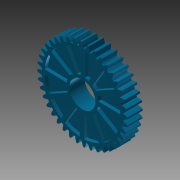
# Autodesk Inventor part: 12-0040_Gear
Saved by Autodesk Inventor 2015 SP1 (Build 190203100, 203)
## iProperties
Category: Gear Kit
Company: Autodesk Inc.
Created: 2014-11-29
Part Number: 12-0040_Gear
Material: Polystyrene, High Impact
Document SubType Name: Modeling
Designer: Matrix
Density: 1.022 g/cm^3
Appearance: Sky Blue Dark
Catalog Web Link: http://matrixrobotics.com/
Vendor: Matrix
Author: Autodesk Inc.
Autodesk Inventor part; units mm, degrees
ref_plane "YZ Plane" through (0, 0, 0) normal (1, 0, 0) x (0, 1, 0)
ref_plane "XZ Plane" through (0, 0, 0) normal (0, 1, 0) x (-1, 0, 0)
sketch "Sketch1" plane through (0, 0, 0) normal (0, 1, 0) x (-1, 0, 0)
  line L0 (9.9681, 15.9078) -> (10.1982, 16.6846)
  arc A0 (10.1982, 16.6846) -> (10.2097, 16.7356) centre (9.8146, 16.7982) ccw
  line L1 (10.2097, 16.7356) -> (10.3968, 17.917)
  arc A1 (10.3968, 17.917) -> (10.2983, 18.1191) centre (10.2032, 17.9477) ccw
  line L2 (9.9086, 18.3351) -> (10.2983, 18.1191)
  arc A2 (9.9086, 18.3351) -> (9.685, 18.3116) centre (9.8136, 18.1636) ccw
  line L3 (9.685, 18.3116) -> (8.7823, 17.5268)
  arc A3 (8.7823, 17.5268) -> (8.7451, 17.49) centre (9.0447, 17.225) ccw
  line L4 (8.7451, 17.49) -> (8.2083, 16.8833)
  arc A4 (8.0902, 16.8594) -> (8.2083, 16.8833) centre (8.1334, 16.9495) ccw
  arc A5 (8.0902, 16.8594) -> (7.4163, 17.1665) centre (0, 0) ccw
  arc A6 (7.3568, 17.2713) -> (7.4163, 17.1665) centre (7.456, 17.2583) ccw
  line L5 (7.3568, 17.2713) -> (7.466, 18.1005)
  line L6 (7.466, 18.1005) -> (7.466, 19.3228)
  arc A7 (7.466, 19.3228) -> (7.337, 19.507) centre (7.27, 19.3228) ccw
  line L7 (7.337, 19.507) -> (6.9184, 19.6594)
  arc A8 (6.9184, 19.6594) -> (6.7012, 19.6012) centre (6.8513, 19.4752) ccw
  line L8 (6.7012, 19.6012) -> (5.9155, 18.6648)
  line L9 (5.9155, 18.6648) -> (5.4661, 17.9595)
  arc A9 (5.3532, 17.9174) -> (5.4661, 17.9595) centre (5.3818, 18.0132) ccw
  arc A10 (5.3532, 17.9174) -> (4.6396, 18.1153) centre (0, 0) ccw
  arc A11 (4.5644, 18.2096) -> (4.6396, 18.1153) centre (4.6644, 18.2122) ccw
  line L10 (4.5644, 18.2096) -> (4.5425, 19.0456)
  line L11 (4.5425, 19.0456) -> (4.3513, 20.2529)
  arc A12 (4.3513, 20.2529) -> (4.1951, 20.4146) centre (4.1577, 20.2222) ccw
  line L12 (4.1951, 20.4146) -> (3.7578, 20.4996)
  arc A13 (3.7578, 20.4996) -> (3.5524, 20.4082) centre (3.7204, 20.3072) ccw
  line L13 (3.5524, 20.4082) -> (2.9228, 19.3604)
  line L14 (2.9228, 19.3604) -> (2.5894, 18.5935)
  arc A14 (2.4844, 18.5342) -> (2.5894, 18.5935) centre (2.4977, 18.6333) ccw
  arc A15 (2.4844, 18.5342) -> (1.7486, 18.6181) centre (0, 0) ccw
  arc A16 (1.6596, 18.6994) -> (1.7486, 18.6181) centre (1.7579, 18.7176) ccw
  line L15 (1.6596, 18.6994) -> (1.5072, 19.5217)
  line L16 (1.5072, 19.5217) -> (1.1295, 20.6842)
  arc A17 (1.1295, 20.6842) -> (0.9499, 20.8195) centre (0.9431, 20.6237) ccw
  line L17 (0.9499, 20.8195) -> (0.5047, 20.8351)
  arc A18 (0.5047, 20.8351) -> (0.3161, 20.7126) centre (0.4978, 20.6392) ccw
  line L18 (0.3161, 20.7126) -> (-0.1418, 19.5793)
  line L19 (-0.1418, 19.5793) -> (-0.3512, 18.7696)
  arc A19 (-0.4456, 18.6947) -> (-0.3512, 18.7696) centre (-0.448, 18.7947) ccw
  arc A20 (-0.4456, 18.6947) -> (-1.1854, 18.6624) centre (0, 0) ccw
  arc A21 (-1.286, 18.7288) -> (-1.1854, 18.6624) centre (-1.1918, 18.7622) ccw
  line L20 (-1.286, 18.7288) -> (-1.5652, 19.5171)
  line L21 (-1.5652, 19.5171) -> (-2.1201, 20.6063)
  arc A22 (-2.1201, 20.6063) -> (-2.3187, 20.7118) centre (-2.2948, 20.5173) ccw
  line L22 (-2.3187, 20.7118) -> (-2.7609, 20.6575)
  arc A23 (-2.7609, 20.6575) -> (-2.9279, 20.5071) centre (-2.737, 20.463) ccw
  line L23 (-2.9279, 20.5071) -> (-3.2029, 19.3161)
  line L24 (-3.2029, 19.3161) -> (-3.2831, 18.4836)
  arc A24 (-3.3646, 18.3948) -> (-3.2831, 18.4836) centre (-3.3826, 18.4932) ccw
  arc A25 (-3.3646, 18.3948) -> (-4.0903, 18.2472) centre (0, 0) ccw
  arc A26 (-4.2, 18.297) -> (-4.0903, 18.2472) centre (-4.1122, 18.3448) ccw
  line L25 (-4.2, 18.297) -> (-4.5991, 19.032)
  line L26 (-4.5991, 19.032) -> (-5.3176, 20.0209)
  arc A27 (-5.3176, 20.0209) -> (-5.5302, 20.0941) centre (-5.4761, 19.9057) ccw
  line L27 (-5.5302, 20.0941) -> (-5.9584, 19.9713)
  arc A28 (-5.9584, 19.9713) -> (-6.0999, 19.7966) centre (-5.9044, 19.7829) ccw
  line L28 (-6.0999, 19.7966) -> (-6.1852, 18.5772)
  line L29 (-6.1852, 18.5772) -> (-6.1341, 17.7425)
  arc A29 (-6.2008, 17.642) -> (-6.1341, 17.7425) centre (-6.2339, 17.7363) ccw
  arc A30 (-6.2008, 17.642) -> (-6.8944, 17.3827) centre (0, 0) ccw
  arc A31 (-7.0106, 17.4147) -> (-6.8944, 17.3827) centre (-6.9313, 17.4756) ccw
  line L30 (-7.0106, 17.4147) -> (-7.5197, 18.0782)
  line L31 (-7.5197, 18.0782) -> (-8.384, 18.9426)
  arc A32 (-8.384, 18.9426) -> (-8.6055, 18.9816) centre (-8.5226, 18.804) ccw
  line L32 (-8.6055, 18.9816) -> (-9.0093, 18.7933)
  arc A33 (-9.0093, 18.7933) -> (-9.1217, 18.5986) centre (-8.9264, 18.6157) ccw
  line L33 (-9.1217, 18.5986) -> (-9.0151, 17.3809)
  line L34 (-9.0151, 17.3809) -> (-8.8341, 16.5644)
  arc A34 (-8.8843, 16.4548) -> (-8.8341, 16.5644) centre (-8.9318, 16.5428) ccw
  arc A35 (-8.8843, 16.4548) -> (-9.5288, 16.0901) centre (0, 0) ccw
  arc A36 (-9.6486, 16.1036) -> (-9.5288, 16.0901) centre (-9.5797, 16.1762) ccw
  line L35 (-9.6486, 16.1036) -> (-10.2552, 16.6793)
  line L36 (-10.2552, 16.6793) -> (-11.2441, 17.3978)
  arc A37 (-11.2441, 17.3978) -> (-11.4689, 17.4017) centre (-11.3593, 17.2392) ccw
  line L37 (-11.4689, 17.4017) -> (-11.8383, 17.1526)
  arc A38 (-11.8383, 17.1526) -> (-11.9188, 16.9427) centre (-11.7287, 16.9901) ccw
  line L38 (-11.9188, 16.9427) -> (-11.6231, 15.7566)
  line L39 (-11.6231, 15.7566) -> (-11.3166, 14.9785)
  arc A39 (-11.349, 14.8624) -> (-11.3166, 14.9785) centre (-11.4097, 14.9419) ccw
  arc A40 (-11.349, 14.8624) -> (-11.9285, 14.4014) centre (0, 0) ccw
  arc A41 (-12.0489, 14.396) -> (-11.9285, 14.4014) centre (-11.9923, 14.4784) ccw
  line L40 (-12.0489, 14.396) -> (-12.7382, 14.8697)
  line L41 (-12.7382, 14.8697) -> (-13.8273, 15.4246)
  arc A42 (-13.8273, 15.4246) -> (-14.0499, 15.3933) centre (-13.9163, 15.25) ccw
  line L42 (-14.0499, 15.3933) -> (-14.3758, 15.0895)
  arc A43 (-14.3758, 15.0895) -> (-14.4225, 14.8696) centre (-14.2421, 14.9461) ccw
  line L43 (-14.4225, 14.8696) -> (-13.9449, 13.7444)
  line L44 (-13.9449, 13.7444) -> (-13.5204, 13.0238)
  arc A44 (-13.5342, 12.9041) -> (-13.5204, 13.0238) centre (-13.6066, 12.9731) ccw
  arc A45 (-13.5342, 12.9041) -> (-14.0345, 12.3581) centre (0, 0) ccw
  arc A46 (-14.1526, 12.3339) -> (-14.0345, 12.3581) centre (-14.1096, 12.4242) ccw
  line L45 (-14.1526, 12.3339) -> (-14.9075, 12.6939)
  line L46 (-14.9075, 12.6939) -> (-16.07, 13.0717)
  arc A47 (-16.07, 13.0717) -> (-16.285, 13.0059) centre (-16.1305, 12.8853) ccw
  line L47 (-16.285, 13.0059) -> (-16.5593, 12.6548)
  arc A48 (-16.5593, 12.6548) -> (-16.5711, 12.4303) centre (-16.4048, 12.5342) ccw
  line L48 (-16.5711, 12.4303) -> (-15.9233, 11.3937)
  line L49 (-15.9233, 11.3937) -> (-15.3914, 10.7484)
  arc A49 (-15.3862, 10.628) -> (-15.3914, 10.7484) centre (-15.4685, 10.6848) ccw
  arc A50 (-15.3862, 10.628) -> (-15.795, 10.0104) centre (0, 0) ccw
  arc A51 (-15.9078, 9.9681) -> (-15.795, 10.0104) centre (-15.8794, 10.064) ccw
  line L50 (-15.9078, 9.9681) -> (-16.7097, 10.2056)
  line L51 (-16.7097, 10.2056) -> (-17.917, 10.3968)
  arc A52 (-17.917, 10.3968) -> (-18.1191, 10.2983) centre (-17.9477, 10.2032) ccw
  line L52 (-18.3351, 9.9086) -> (-18.1191, 10.2983)
  arc A53 (-18.3351, 9.9086) -> (-18.3116, 9.685) centre (-18.1636, 9.8136) ccw
  line L53 (-18.3116, 9.685) -> (-17.5096, 8.7625)
  line L54 (-17.5096, 8.7625) -> (-16.8833, 8.2083)
  arc A54 (-16.8594, 8.0902) -> (-16.8833, 8.2083) centre (-16.9495, 8.1334) ccw
  arc A55 (-16.8594, 8.0902) -> (-17.1665, 7.4163) centre (0, 0) ccw
  arc A56 (-17.2713, 7.3568) -> (-17.1665, 7.4163) centre (-17.2583, 7.456) ccw
  line L55 (-17.2713, 7.3568) -> (-18.1005, 7.466)
  line L56 (-18.1005, 7.466) -> (-19.3228, 7.466)
  arc A57 (-19.3228, 7.466) -> (-19.507, 7.337) centre (-19.3228, 7.27) ccw
  line L57 (-19.507, 7.337) -> (-19.6594, 6.9184)
  arc A58 (-19.6594, 6.9184) -> (-19.6012, 6.7012) centre (-19.4752, 6.8513) ccw
  line L58 (-19.6012, 6.7012) -> (-18.6648, 5.9155)
  line L59 (-18.6648, 5.9155) -> (-17.9595, 5.4661)
  arc A59 (-17.9174, 5.3532) -> (-17.9595, 5.4661) centre (-18.0132, 5.3818) ccw
  arc A60 (-17.9174, 5.3532) -> (-18.1153, 4.6396) centre (0, 0) ccw
  arc A61 (-18.2096, 4.5644) -> (-18.1153, 4.6396) centre (-18.2122, 4.6644) ccw
  line L60 (-18.2096, 4.5644) -> (-19.0456, 4.5425)
  line L61 (-19.0456, 4.5425) -> (-20.2529, 4.3513)
  arc A62 (-20.2529, 4.3513) -> (-20.4146, 4.1951) centre (-20.2222, 4.1577) ccw
  line L62 (-20.4146, 4.1951) -> (-20.4996, 3.7578)
  arc A63 (-20.4996, 3.7578) -> (-20.4082, 3.5524) centre (-20.3072, 3.7204) ccw
  line L63 (-20.4082, 3.5524) -> (-19.3604, 2.9228)
  line L64 (-19.3604, 2.9228) -> (-18.5935, 2.5894)
  arc A64 (-18.5342, 2.4844) -> (-18.5935, 2.5894) centre (-18.6333, 2.4977) ccw
  arc A65 (-18.5342, 2.4844) -> (-18.6181, 1.7486) centre (0, 0) ccw
  arc A66 (-18.6994, 1.6596) -> (-18.6181, 1.7486) centre (-18.7176, 1.7579) ccw
  line L65 (-18.6994, 1.6596) -> (-19.5217, 1.5072)
  line L66 (-19.5217, 1.5072) -> (-20.6842, 1.1295)
  arc A67 (-20.6842, 1.1295) -> (-20.8195, 0.9499) centre (-20.6237, 0.9431) ccw
  line L67 (-20.8195, 0.9499) -> (-20.8351, 0.5047)
  arc A68 (-20.8351, 0.5047) -> (-20.7126, 0.3161) centre (-20.6392, 0.4978) ccw
  line L68 (-20.7126, 0.3161) -> (-19.5793, -0.1418)
  line L69 (-19.5793, -0.1418) -> (-18.7696, -0.3512)
  arc A69 (-18.6947, -0.4456) -> (-18.7696, -0.3512) centre (-18.7947, -0.448) ccw
  arc A70 (-18.6947, -0.4456) -> (-18.6624, -1.1854) centre (0, 0) ccw
  arc A71 (-18.7288, -1.286) -> (-18.6624, -1.1854) centre (-18.7622, -1.1918) ccw
  line L70 (-18.7288, -1.286) -> (-19.5171, -1.5652)
  line L71 (-19.5171, -1.5652) -> (-20.6063, -2.1201)
  arc A72 (-20.6063, -2.1201) -> (-20.7118, -2.3187) centre (-20.5173, -2.2948) ccw
  line L72 (-20.7118, -2.3187) -> (-20.6575, -2.7609)
  arc A73 (-20.6575, -2.7609) -> (-20.5071, -2.9279) centre (-20.463, -2.737) ccw
  line L73 (-20.5071, -2.9279) -> (-19.3161, -3.2029)
  line L74 (-19.3161, -3.2029) -> (-18.4836, -3.2831)
  arc A74 (-18.3948, -3.3646) -> (-18.4836, -3.2831) centre (-18.4932, -3.3826) ccw
  arc A75 (-18.3948, -3.3646) -> (-18.2472, -4.0903) centre (0, 0) ccw
  arc A76 (-18.297, -4.2) -> (-18.2472, -4.0903) centre (-18.3448, -4.1122) ccw
  line L75 (-18.297, -4.2) -> (-19.032, -4.5991)
  line L76 (-19.032, -4.5991) -> (-20.0209, -5.3176)
  arc A77 (-20.0209, -5.3176) -> (-20.0941, -5.5302) centre (-19.9057, -5.4761) ccw
  line L77 (-20.0941, -5.5302) -> (-19.9713, -5.9584)
  arc A78 (-19.9713, -5.9584) -> (-19.7966, -6.0999) centre (-19.7829, -5.9044) ccw
  line L78 (-19.7966, -6.0999) -> (-18.5772, -6.1852)
  line L79 (-18.5772, -6.1852) -> (-17.7425, -6.1341)
  arc A79 (-17.642, -6.2008) -> (-17.7425, -6.1341) centre (-17.7363, -6.2339) ccw
  arc A80 (-17.642, -6.2008) -> (-17.3827, -6.8944) centre (0, 0) ccw
  arc A81 (-17.4147, -7.0106) -> (-17.3827, -6.8944) centre (-17.4756, -6.9313) ccw
  line L80 (-17.4147, -7.0106) -> (-18.0782, -7.5197)
  line L81 (-18.0782, -7.5197) -> (-18.9426, -8.384)
  arc A82 (-18.9426, -8.384) -> (-18.9816, -8.6055) centre (-18.804, -8.5226) ccw
  line L82 (-18.9816, -8.6055) -> (-18.7933, -9.0093)
  arc A83 (-18.7933, -9.0093) -> (-18.5986, -9.1217) centre (-18.6157, -8.9264) ccw
  line L83 (-18.5986, -9.1217) -> (-17.3809, -9.0151)
  line L84 (-17.3809, -9.0151) -> (-16.5644, -8.8341)
  arc A84 (-16.4548, -8.8843) -> (-16.5644, -8.8341) centre (-16.5428, -8.9318) ccw
  arc A85 (-16.4548, -8.8843) -> (-16.0901, -9.5288) centre (0, 0) ccw
  arc A86 (-16.1036, -9.6486) -> (-16.0901, -9.5288) centre (-16.1762, -9.5797) ccw
  line L85 (-16.1036, -9.6486) -> (-16.6793, -10.2552)
  line L86 (-16.6793, -10.2552) -> (-17.3978, -11.2441)
  arc A87 (-17.3978, -11.2441) -> (-17.4017, -11.4689) centre (-17.2392, -11.3593) ccw
  line L87 (-17.4017, -11.4689) -> (-17.1526, -11.8383)
  arc A88 (-17.1526, -11.8383) -> (-16.9427, -11.9188) centre (-16.9901, -11.7287) ccw
  line L88 (-16.9427, -11.9188) -> (-15.7566, -11.6231)
  line L89 (-15.7566, -11.6231) -> (-14.9785, -11.3166)
  arc A89 (-14.8624, -11.349) -> (-14.9785, -11.3166) centre (-14.9419, -11.4097) ccw
  arc A90 (-14.8624, -11.349) -> (-14.4014, -11.9285) centre (0, 0) ccw
  arc A91 (-14.396, -12.0489) -> (-14.4014, -11.9285) centre (-14.4784, -11.9923) ccw
  line L90 (-14.396, -12.0489) -> (-14.8697, -12.7382)
  line L91 (-14.8697, -12.7382) -> (-15.4246, -13.8273)
  arc A92 (-15.4246, -13.8273) -> (-15.3933, -14.0499) centre (-15.25, -13.9163) ccw
  line L92 (-15.3933, -14.0499) -> (-15.0895, -14.3758)
  arc A93 (-15.0895, -14.3758) -> (-14.8696, -14.4225) centre (-14.9461, -14.2421) ccw
  line L93 (-14.8696, -14.4225) -> (-13.7444, -13.9449)
  line L94 (-13.7444, -13.9449) -> (-13.0238, -13.5204)
  arc A94 (-12.9041, -13.5342) -> (-13.0238, -13.5204) centre (-12.9731, -13.6066) ccw
  arc A95 (-12.9041, -13.5342) -> (-12.3581, -14.0345) centre (0, 0) ccw
  arc A96 (-12.3339, -14.1526) -> (-12.3581, -14.0345) centre (-12.4242, -14.1096) ccw
  line L95 (-12.3339, -14.1526) -> (-12.6939, -14.9075)
  line L96 (-12.6939, -14.9075) -> (-13.0717, -16.07)
  arc A97 (-13.0717, -16.07) -> (-13.0059, -16.285) centre (-12.8853, -16.1305) ccw
  line L97 (-13.0059, -16.285) -> (-12.6548, -16.5593)
  arc A98 (-12.6548, -16.5593) -> (-12.4303, -16.5711) centre (-12.5342, -16.4048) ccw
  line L98 (-12.4303, -16.5711) -> (-11.3937, -15.9233)
  line L99 (-11.3937, -15.9233) -> (-10.7484, -15.3914)
  arc A99 (-10.628, -15.3862) -> (-10.7484, -15.3914) centre (-10.6848, -15.4685) ccw
  arc A100 (-10.628, -15.3862) -> (-10.0104, -15.795) centre (0, 0) ccw
  arc A101 (-9.9681, -15.9078) -> (-10.0104, -15.795) centre (-10.064, -15.8794) ccw
  line L100 (-9.9681, -15.9078) -> (-10.2056, -16.7097)
  line L101 (-10.2056, -16.7097) -> (-10.3968, -17.917)
  arc A102 (-10.3968, -17.917) -> (-10.2983, -18.1191) centre (-10.2032, -17.9477) ccw
  line L102 (-9.9086, -18.3351) -> (-10.2983, -18.1191)
  arc A103 (-9.9086, -18.3351) -> (-9.685, -18.3116) centre (-9.8136, -18.1636) ccw
  line L103 (-9.685, -18.3116) -> (-8.7625, -17.5096)
  line L104 (-8.7625, -17.5096) -> (-8.2083, -16.8833)
  arc A104 (-8.0902, -16.8594) -> (-8.2083, -16.8833) centre (-8.1334, -16.9495) ccw
  arc A105 (-8.0902, -16.8594) -> (-7.4163, -17.1665) centre (0, 0) ccw
  arc A106 (-7.3568, -17.2713) -> (-7.4163, -17.1665) centre (-7.456, -17.2583) ccw
  line L105 (-7.3568, -17.2713) -> (-7.466, -18.1005)
  line L106 (-7.466, -18.1005) -> (-7.466, -19.3228)
  arc A107 (-7.466, -19.3228) -> (-7.337, -19.507) centre (-7.27, -19.3228) ccw
  line L107 (-7.337, -19.507) -> (-6.9184, -19.6594)
  arc A108 (-6.9184, -19.6594) -> (-6.7012, -19.6012) centre (-6.8513, -19.4752) ccw
  line L108 (-6.7012, -19.6012) -> (-5.9155, -18.6648)
  line L109 (-5.9155, -18.6648) -> (-5.4661, -17.9595)
  arc A109 (-5.3532, -17.9174) -> (-5.4661, -17.9595) centre (-5.3818, -18.0132) ccw
  arc A110 (-5.3532, -17.9174) -> (-4.6396, -18.1153) centre (0, 0) ccw
  arc A111 (-4.5644, -18.2096) -> (-4.6396, -18.1153) centre (-4.6644, -18.2122) ccw
  line L110 (-4.5644, -18.2096) -> (-4.5425, -19.0456)
  line L111 (-4.5425, -19.0456) -> (-4.3513, -20.2529)
  arc A112 (-4.3513, -20.2529) -> (-4.1951, -20.4146) centre (-4.1577, -20.2222) ccw
  line L112 (-4.1951, -20.4146) -> (-3.7578, -20.4996)
  arc A113 (-3.7578, -20.4996) -> (-3.5524, -20.4082) centre (-3.7204, -20.3072) ccw
  line L113 (-3.5524, -20.4082) -> (-2.9228, -19.3604)
  line L114 (-2.9228, -19.3604) -> (-2.5894, -18.5935)
  arc A114 (-2.4844, -18.5342) -> (-2.5894, -18.5935) centre (-2.4977, -18.6333) ccw
  arc A115 (-2.4844, -18.5342) -> (-1.7486, -18.6181) centre (0, 0) ccw
  arc A116 (-1.6596, -18.6994) -> (-1.7486, -18.6181) centre (-1.7579, -18.7176) ccw
  line L115 (-1.6596, -18.6994) -> (-1.5072, -19.5217)
  line L116 (-1.5072, -19.5217) -> (-1.1295, -20.6842)
  arc A117 (-1.1295, -20.6842) -> (-0.9499, -20.8195) centre (-0.9431, -20.6237) ccw
  line L117 (-0.9499, -20.8195) -> (-0.5047, -20.8351)
  arc A118 (-0.5047, -20.8351) -> (-0.3161, -20.7126) centre (-0.4978, -20.6392) ccw
  line L118 (-0.3161, -20.7126) -> (0.1418, -19.5793)
  line L119 (0.1418, -19.5793) -> (0.3512, -18.7696)
  arc A119 (0.4456, -18.6947) -> (0.3512, -18.7696) centre (0.448, -18.7947) ccw
  arc A120 (0.4456, -18.6947) -> (1.1854, -18.6624) centre (0, 0) ccw
  arc A121 (1.286, -18.7288) -> (1.1854, -18.6624) centre (1.1918, -18.7622) ccw
  line L120 (1.286, -18.7288) -> (1.5652, -19.5171)
  line L121 (1.5652, -19.5171) -> (2.1201, -20.6063)
  arc A122 (2.1201, -20.6063) -> (2.3187, -20.7118) centre (2.2948, -20.5173) ccw
  line L122 (2.3187, -20.7118) -> (2.7609, -20.6575)
  arc A123 (2.7609, -20.6575) -> (2.9279, -20.5071) centre (2.737, -20.463) ccw
  line L123 (2.9279, -20.5071) -> (3.2029, -19.3161)
  line L124 (3.2029, -19.3161) -> (3.2831, -18.4836)
  arc A124 (3.3646, -18.3948) -> (3.2831, -18.4836) centre (3.3826, -18.4932) ccw
  arc A125 (3.3646, -18.3948) -> (4.0903, -18.2472) centre (0, 0) ccw
  arc A126 (4.2, -18.297) -> (4.0903, -18.2472) centre (4.1122, -18.3448) ccw
  line L125 (4.2, -18.297) -> (4.5991, -19.032)
  line L126 (4.5991, -19.032) -> (5.3176, -20.0209)
  arc A127 (5.3176, -20.0209) -> (5.5302, -20.0941) centre (5.4761, -19.9057) ccw
  line L127 (5.5302, -20.0941) -> (5.9584, -19.9713)
  arc A128 (5.9584, -19.9713) -> (6.0999, -19.7966) centre (5.9044, -19.7829) ccw
  line L128 (6.0999, -19.7966) -> (6.1852, -18.5772)
  line L129 (6.1852, -18.5772) -> (6.1341, -17.7425)
  arc A129 (6.2008, -17.642) -> (6.1341, -17.7425) centre (6.2339, -17.7363) ccw
  arc A130 (6.2008, -17.642) -> (6.8944, -17.3827) centre (0, 0) ccw
  arc A131 (7.0106, -17.4147) -> (6.8944, -17.3827) centre (6.9313, -17.4756) ccw
  line L130 (7.0106, -17.4147) -> (7.5197, -18.0782)
  line L131 (7.5197, -18.0782) -> (8.384, -18.9426)
  arc A132 (8.384, -18.9426) -> (8.6055, -18.9816) centre (8.5226, -18.804) ccw
  line L132 (8.6055, -18.9816) -> (9.0093, -18.7933)
  arc A133 (9.0093, -18.7933) -> (9.1217, -18.5986) centre (8.9264, -18.6157) ccw
  line L133 (9.1217, -18.5986) -> (9.0151, -17.3809)
  line L134 (9.0151, -17.3809) -> (8.8341, -16.5644)
  arc A134 (8.8843, -16.4548) -> (8.8341, -16.5644) centre (8.9318, -16.5428) ccw
  arc A135 (8.8843, -16.4548) -> (9.5288, -16.0901) centre (0, 0) ccw
  arc A136 (9.6486, -16.1036) -> (9.5288, -16.0901) centre (9.5797, -16.1762) ccw
  line L135 (9.6486, -16.1036) -> (10.2552, -16.6793)
  line L136 (10.2552, -16.6793) -> (11.2441, -17.3978)
  arc A137 (11.2441, -17.3978) -> (11.4689, -17.4017) centre (11.3593, -17.2392) ccw
  line L137 (11.4689, -17.4017) -> (11.8383, -17.1526)
  arc A138 (11.8383, -17.1526) -> (11.9188, -16.9427) centre (11.7287, -16.9901) ccw
  line L138 (11.9188, -16.9427) -> (11.6231, -15.7566)
  line L139 (11.6231, -15.7566) -> (11.3166, -14.9785)
  arc A139 (11.349, -14.8624) -> (11.3166, -14.9785) centre (11.4097, -14.9419) ccw
  arc A140 (11.349, -14.8624) -> (11.9285, -14.4014) centre (0, 0) ccw
  arc A141 (12.0489, -14.396) -> (11.9285, -14.4014) centre (11.9923, -14.4784) ccw
  line L140 (12.0489, -14.396) -> (12.7382, -14.8697)
  line L141 (12.7382, -14.8697) -> (13.8273, -15.4246)
  arc A142 (13.8273, -15.4246) -> (14.0499, -15.3933) centre (13.9163, -15.25) ccw
  line L142 (14.0499, -15.3933) -> (14.3758, -15.0895)
  arc A143 (14.3758, -15.0895) -> (14.4225, -14.8696) centre (14.2421, -14.9461) ccw
  line L143 (14.4225, -14.8696) -> (13.9449, -13.7444)
  line L144 (13.9449, -13.7444) -> (13.5204, -13.0238)
  arc A144 (13.5342, -12.9041) -> (13.5204, -13.0238) centre (13.6066, -12.9731) ccw
  arc A145 (13.5342, -12.9041) -> (14.0345, -12.3581) centre (0, 0) ccw
  arc A146 (14.1526, -12.3339) -> (14.0345, -12.3581) centre (14.1096, -12.4242) ccw
  line L145 (14.1526, -12.3339) -> (14.9075, -12.6939)
  line L146 (14.9075, -12.6939) -> (16.07, -13.0717)
  arc A147 (16.07, -13.0717) -> (16.285, -13.0059) centre (16.1305, -12.8853) ccw
  line L147 (16.285, -13.0059) -> (16.5593, -12.6548)
  arc A148 (16.5593, -12.6548) -> (16.5711, -12.4303) centre (16.4048, -12.5342) ccw
  line L148 (16.5711, -12.4303) -> (15.9233, -11.3937)
  line L149 (15.9233, -11.3937) -> (15.3914, -10.7484)
  arc A149 (15.3862, -10.628) -> (15.3914, -10.7484) centre (15.4685, -10.6848) ccw
  arc A150 (15.3862, -10.628) -> (15.795, -10.0104) centre (0, 0) ccw
  arc A151 (15.9078, -9.9681) -> (15.795, -10.0104) centre (15.8794, -10.064) ccw
  line L150 (15.9078, -9.9681) -> (16.7097, -10.2056)
  line L151 (16.7097, -10.2056) -> (17.917, -10.3968)
  arc A152 (17.917, -10.3968) -> (18.1191, -10.2983) centre (17.9477, -10.2032) ccw
  line L152 (18.3351, -9.9086) -> (18.1191, -10.2983)
  arc A153 (18.3351, -9.9086) -> (18.3116, -9.685) centre (18.1636, -9.8136) ccw
  line L153 (18.3116, -9.685) -> (17.5096, -8.7625)
  line L154 (17.5096, -8.7625) -> (16.8833, -8.2083)
  arc A154 (16.8594, -8.0902) -> (16.8833, -8.2083) centre (16.9495, -8.1334) ccw
  arc A155 (16.8594, -8.0902) -> (17.1665, -7.4163) centre (0, 0) ccw
  arc A156 (17.2713, -7.3568) -> (17.1665, -7.4163) centre (17.2583, -7.456) ccw
  line L155 (17.2713, -7.3568) -> (18.1005, -7.466)
  line L156 (18.1005, -7.466) -> (19.3228, -7.466)
  arc A157 (19.3228, -7.466) -> (19.507, -7.337) centre (19.3228, -7.27) ccw
  line L157 (19.507, -7.337) -> (19.6594, -6.9184)
  arc A158 (19.6594, -6.9184) -> (19.6012, -6.7012) centre (19.4752, -6.8513) ccw
  line L158 (19.6012, -6.7012) -> (18.6648, -5.9155)
  line L159 (18.6648, -5.9155) -> (17.9595, -5.4661)
  arc A159 (17.9174, -5.3532) -> (17.9595, -5.4661) centre (18.0132, -5.3818) ccw
  arc A160 (17.9174, -5.3532) -> (18.1153, -4.6396) centre (0, 0) ccw
  arc A161 (18.2096, -4.5644) -> (18.1153, -4.6396) centre (18.2122, -4.6644) ccw
  line L160 (18.2096, -4.5644) -> (19.0456, -4.5425)
  line L161 (19.0456, -4.5425) -> (20.2529, -4.3513)
  arc A162 (20.2529, -4.3513) -> (20.4146, -4.1951) centre (20.2222, -4.1577) ccw
  line L162 (20.4146, -4.1951) -> (20.4996, -3.7578)
  arc A163 (20.4996, -3.7578) -> (20.4082, -3.5524) centre (20.3072, -3.7204) ccw
  line L163 (20.4082, -3.5524) -> (19.3604, -2.9228)
  line L164 (19.3604, -2.9228) -> (18.5935, -2.5894)
  arc A164 (18.5342, -2.4844) -> (18.5935, -2.5894) centre (18.6333, -2.4977) ccw
  arc A165 (18.5342, -2.4844) -> (18.6181, -1.7486) centre (0, 0) ccw
  arc A166 (18.6994, -1.6596) -> (18.6181, -1.7486) centre (18.7176, -1.7579) ccw
  line L165 (18.6994, -1.6596) -> (19.5217, -1.5072)
  line L166 (19.5217, -1.5072) -> (20.6842, -1.1295)
  arc A167 (20.6842, -1.1295) -> (20.8195, -0.9499) centre (20.6237, -0.9431) ccw
  line L167 (20.8195, -0.9499) -> (20.8351, -0.5047)
  arc A168 (20.8351, -0.5047) -> (20.7126, -0.3161) centre (20.6392, -0.4978) ccw
  line L168 (20.7126, -0.3161) -> (19.5793, 0.1418)
  line L169 (19.5793, 0.1418) -> (18.7696, 0.3512)
  arc A169 (18.6947, 0.4456) -> (18.7696, 0.3512) centre (18.7947, 0.448) ccw
  arc A170 (18.6947, 0.4456) -> (18.6624, 1.1854) centre (0, 0) ccw
  arc A171 (18.7288, 1.286) -> (18.6624, 1.1854) centre (18.7622, 1.1918) ccw
  line L170 (18.7288, 1.286) -> (19.5171, 1.5652)
  line L171 (19.5171, 1.5652) -> (20.6063, 2.1201)
  arc A172 (20.6063, 2.1201) -> (20.7118, 2.3187) centre (20.5173, 2.2948) ccw
  line L172 (20.7118, 2.3187) -> (20.6575, 2.7609)
  arc A173 (20.6575, 2.7609) -> (20.5071, 2.9279) centre (20.463, 2.737) ccw
  line L173 (20.5071, 2.9279) -> (19.3161, 3.2029)
  line L174 (19.3161, 3.2029) -> (18.4836, 3.2831)
  arc A174 (18.3948, 3.3646) -> (18.4836, 3.2831) centre (18.4932, 3.3826) ccw
  arc A175 (18.3948, 3.3646) -> (18.2472, 4.0903) centre (0, 0) ccw
  arc A176 (18.297, 4.2) -> (18.2472, 4.0903) centre (18.3448, 4.1122) ccw
  line L175 (18.297, 4.2) -> (19.032, 4.5991)
  line L176 (19.032, 4.5991) -> (20.0209, 5.3176)
  arc A177 (20.0209, 5.3176) -> (20.0941, 5.5302) centre (19.9057, 5.4761) ccw
  line L177 (20.0941, 5.5302) -> (19.9713, 5.9584)
  arc A178 (19.9713, 5.9584) -> (19.7966, 6.0999) centre (19.7829, 5.9044) ccw
  line L178 (19.7966, 6.0999) -> (18.5772, 6.1852)
  line L179 (18.5772, 6.1852) -> (17.7425, 6.1341)
  arc A179 (17.642, 6.2008) -> (17.7425, 6.1341) centre (17.7363, 6.2339) ccw
  arc A180 (17.642, 6.2008) -> (17.3827, 6.8944) centre (0, 0) ccw
  arc A181 (17.4147, 7.0106) -> (17.3827, 6.8944) centre (17.4756, 6.9313) ccw
  line L180 (17.4147, 7.0106) -> (18.0782, 7.5197)
  line L181 (18.0782, 7.5197) -> (18.9426, 8.384)
  arc A182 (18.9426, 8.384) -> (18.9816, 8.6055) centre (18.804, 8.5226) ccw
  line L182 (18.9816, 8.6055) -> (18.7933, 9.0093)
  arc A183 (18.7933, 9.0093) -> (18.5986, 9.1217) centre (18.6157, 8.9264) ccw
  line L183 (18.5986, 9.1217) -> (17.3809, 9.0151)
  line L184 (17.3809, 9.0151) -> (16.5644, 8.8341)
  arc A184 (16.4548, 8.8843) -> (16.5644, 8.8341) centre (16.5428, 8.9318) ccw
  arc A185 (16.4548, 8.8843) -> (16.0901, 9.5288) centre (0, 0) ccw
  arc A186 (16.1036, 9.6486) -> (16.0901, 9.5288) centre (16.1762, 9.5797) ccw
  line L185 (16.1036, 9.6486) -> (16.6793, 10.2552)
  line L186 (16.6793, 10.2552) -> (17.3978, 11.2441)
  arc A187 (17.3978, 11.2441) -> (17.4017, 11.4689) centre (17.2392, 11.3593) ccw
  line L187 (17.4017, 11.4689) -> (17.1526, 11.8383)
  arc A188 (17.1526, 11.8383) -> (16.9427, 11.9188) centre (16.9901, 11.7287) ccw
  line L188 (16.9427, 11.9188) -> (15.7566, 11.6231)
  line L189 (15.7566, 11.6231) -> (14.9785, 11.3166)
  arc A189 (14.8624, 11.349) -> (14.9785, 11.3166) centre (14.9419, 11.4097) ccw
  arc A190 (14.8624, 11.349) -> (14.4014, 11.9285) centre (0, 0) ccw
  arc A191 (14.396, 12.0489) -> (14.4014, 11.9285) centre (14.4784, 11.9923) ccw
  line L190 (14.396, 12.0489) -> (14.8697, 12.7382)
  line L191 (14.8697, 12.7382) -> (15.4246, 13.8273)
  arc A192 (15.4246, 13.8273) -> (15.3933, 14.0499) centre (15.25, 13.9163) ccw
  line L192 (15.3933, 14.0499) -> (15.0895, 14.3758)
  arc A193 (15.0895, 14.3758) -> (14.8696, 14.4225) centre (14.9461, 14.2421) ccw
  line L193 (14.8696, 14.4225) -> (13.7444, 13.9449)
  line L194 (13.7444, 13.9449) -> (13.0238, 13.5204)
  arc A194 (12.9041, 13.5342) -> (13.0238, 13.5204) centre (12.9731, 13.6066) ccw
  arc A195 (12.9041, 13.5342) -> (12.3581, 14.0345) centre (0, 0) ccw
  arc A196 (12.3339, 14.1526) -> (12.3581, 14.0345) centre (12.4242, 14.1096) ccw
  line L195 (12.3339, 14.1526) -> (12.6939, 14.9075)
  line L196 (12.6939, 14.9075) -> (13.0717, 16.07)
  arc A197 (13.0717, 16.07) -> (13.0059, 16.285) centre (12.8853, 16.1305) ccw
  line L197 (13.0059, 16.285) -> (12.6548, 16.5593)
  arc A198 (12.6548, 16.5593) -> (12.4303, 16.5711) centre (12.5342, 16.4048) ccw
  line L198 (12.4303, 16.5711) -> (11.3937, 15.9233)
  line L199 (11.3937, 15.9233) -> (10.7484, 15.3914)
  arc A199 (10.628, 15.3862) -> (10.7484, 15.3914) centre (10.6848, 15.4685) ccw
  arc A200 (10.628, 15.3862) -> (10.0104, 15.795) centre (0, 0) ccw
  arc A201 (9.9681, 15.9078) -> (10.0104, 15.795) centre (10.064, 15.8794) ccw
  arc A202 (-15.7656, 7.5957) -> (-17.4862, 0.6949) centre (0, 0) ccw
  line L200 (-15.7656, 7.5957) -> (-6.8379, 2.647)
  arc A203 (-6.8379, 2.647) -> (-7.2802, 0.8731) centre (0, 0) ccw
  line L201 (-7.2802, 0.8731) -> (-17.4862, 0.6949)
  arc A204 (-14.4609, -9.8556) -> (-9.3449, -14.796) centre (0, 0) ccw
  line L202 (-14.4609, -9.8556) -> (-5.7113, -4.5983)
  arc A205 (-5.7113, -4.5983) -> (-4.3962, -5.8683) centre (0, 0) ccw
  line L203 (-9.3449, -14.796) -> (-4.3962, -5.8683)
  arc A206 (1.3048, -17.4513) -> (8.1413, -15.491) centre (0, 0) ccw
  line L204 (1.3048, -17.4513) -> (1.1266, -7.2453)
  arc A207 (1.1266, -7.2453) -> (2.884, -6.7414) centre (0, 0) ccw
  line L205 (2.884, -6.7414) -> (8.1413, -15.491)
  arc A208 (15.7656, -7.5957) -> (17.4862, -0.6949) centre (0, 0) ccw
  line L206 (15.7656, -7.5957) -> (6.8379, -2.647)
  arc A209 (6.8379, -2.647) -> (7.2802, -0.8731) centre (0, 0) ccw
  line L207 (7.2802, -0.8731) -> (17.4862, -0.6949)
  arc A210 (14.4609, 9.8556) -> (9.3449, 14.796) centre (0, 0) ccw
  line L208 (14.4609, 9.8556) -> (5.7113, 4.5983)
  arc A211 (5.7113, 4.5983) -> (4.3962, 5.8683) centre (0, 0) ccw
  line L209 (9.3449, 14.796) -> (4.3962, 5.8683)
  arc A212 (-1.3048, 17.4513) -> (-8.1413, 15.491) centre (0, 0) ccw
  line L210 (-1.3048, 17.4513) -> (-1.1266, 7.2453)
  arc A213 (-1.1266, 7.2453) -> (-2.884, 6.7414) centre (0, 0) ccw
  line L211 (-2.884, 6.7414) -> (-8.1413, 15.491)
  circle A214 centre (0, 0) radius 6
  arc A215 (7.5957, 15.7656) -> (0.6949, 17.4862) centre (0, 0) ccw
  line L212 (7.5957, 15.7656) -> (2.647, 6.8379)
  arc A216 (2.647, 6.8379) -> (0.8731, 7.2802) centre (0, 0) ccw
  line L213 (0.8731, 7.2802) -> (0.6949, 17.4862)
  arc A217 (17.4513, 1.3048) -> (15.491, 8.1413) centre (0, 0) ccw
  line L214 (17.4513, 1.3048) -> (7.2453, 1.1266)
  arc A218 (7.2453, 1.1266) -> (6.7414, 2.884) centre (0, 0) ccw
  line L215 (6.7414, 2.884) -> (15.491, 8.1413)
  arc A219 (9.8556, -14.4609) -> (14.796, -9.3449) centre (0, 0) ccw
  line L216 (9.8556, -14.4609) -> (4.5983, -5.7113)
  arc A220 (4.5983, -5.7113) -> (5.8683, -4.3962) centre (0, 0) ccw
  line L217 (14.796, -9.3449) -> (5.8683, -4.3962)
  arc A221 (-7.5957, -15.7656) -> (-0.6949, -17.4862) centre (0, 0) ccw
  line L218 (-7.5957, -15.7656) -> (-2.647, -6.8379)
  arc A222 (-2.647, -6.8379) -> (-0.8731, -7.2802) centre (0, 0) ccw
  line L219 (-0.8731, -7.2802) -> (-0.6949, -17.4862)
  arc A223 (-17.4513, -1.3048) -> (-15.491, -8.1413) centre (0, 0) ccw
  line L220 (-17.4513, -1.3048) -> (-7.2453, -1.1266)
  arc A224 (-7.2453, -1.1266) -> (-6.7414, -2.884) centre (0, 0) ccw
  line L221 (-6.7414, -2.884) -> (-15.491, -8.1413)
  arc A225 (-9.8556, 14.4609) -> (-14.796, 9.3449) centre (0, 0) ccw
  line L222 (-9.8556, 14.4609) -> (-4.5983, 5.7113)
  arc A226 (-4.5983, 5.7113) -> (-5.8683, 4.3962) centre (0, 0) ccw
  line L223 (-14.796, 9.3449) -> (-5.8683, 4.3962)
  point P0 (0, 0)
  constraints: 452 point on circle, 448 end point, 227 centre point
extrude "Extrusion1" add sketch "Sketch1" against normal blind 7 contours A201 A200 A199 L199 L198 A198 L197 A197 L196 L195 A196 A195 A194 L194 L193 A193 L192 A192 L191 L190 A191 A190 A189 L189 L188 A188 L187 A187 L186 L185 A186 A185 A184 L184 L183 A183 L182 A182 L181 L180 A181 A180 A179 L179 L178 A178 L177 A177 L176 L175 A176 A175 A174 L174 L173 A173 L172 A172 L171 L170 A171 A170 A169 L169 L168 A168 L167 A167 L166 L165 A166 A165 A164 L164 L163 A163 L162 A162 L161 L160 A161 A160 A159 L159 L158 A158 L157 A157 L156 L155 A156 A155 A154 L154 L153 A153 L152 A152 L151 L150 A151 A150 A149 L149 L148 A148 L147 A147 L146 L145 A146 A145 A144 L144 L143 A143 L142 A142 L141 L140 A141 A140 A139 L139 L138 A138 L137 A137 L136 L135 A136 A135 A134 L134 L133 A133 L132 A132 L131 L130 A131 A130 A129 L129 L128 A128 L127 A127 L126 L125 A126 A125 A124 L124 L123 A123 L122 A122 L121 L120 A121 A120 A119 L119 L118 A118 L117 A117 L116 L115 A116 A115 A114 L114 L113 A113 L112 A112 L111 L110 A111 A110 A109 L109 L108 A108 L107 A107 L106 L105 A106 A105 A104 L104 L103 A103 L102 A102 L101 L100 A101 A100 A99 L99 L98 A98 L97 A97 L96 L95 A96 A95 A94 L94 L93 A93 L92 A92 L91 L90 A91 A90 A89 L89 L88 A88 L87 A87 L86 L85 A86 A85 A84 L84 L83 A83 L82 A82 L81 L80 A81 A80 A79 L79 L78 A78 L77 A77 L76 L75 A76 A75 A74 L74 L73 A73 L72 A72 L71 L70 A71 A70 A69 L69 L68 A68 L67 A67 L66 L65 A66 A65 A64 L64 L63 A63 L62 A62 L61 L60 A61 A60 A59 L59 L58 A58 L57 A57 L56 L55 A56 A55 A54 L54 L53 A53 L52 A52 L51 L50 A51 A50 A49 L49 L48 A48 L47 A47 L46 L45 A46 A45 A44 L44 L43 A43 L42 A42 L41 L40 A41 A40 A39 L39 L38 A38 L37 A37 L36 L35 A36 A35 A34 L34 L33 A33 L32 A32 L31 L30 A31 A30 A29 L29 L28 A28 L27 A27 L26 L25 A26 A25 A24 L24 L23 A23 L22 A22 L21 L20 A21 A20 A19 L19 L18 A18 L17 A17 L16 L15 A16 A15 A14 L14 L13 A13 L12 A12 L11 L10 A11 A10 A9 L9 L8 A8 L7 A7 L6 L5 A6 A5 A4 L4 A3 L3 A2 L2 A1 L1 A0 L0 | L200 A203 L201 A202 | L202 A205 L203 A204 | L204 A207 L205 A206 | L206 A209 L207 A208 | L208 A211 L209 A210 | L210 A213 L211 A212 | L212 A216 L213 A215 | L214 A218 L215 A217 | L216 A220 L217 A219 | L218 A222 L219 A221 | L220 A224 L221 A223 | L222 A226 L223 A225
extrude "Extrusion2" cut sketch "Sketch1" against normal blind 1.5 contours L200 A203 L201 A202 | L202 A205 L203 A204 | L204 A207 L205 A206 | L206 A209 L207 A208 | L208 A211 L209 A210 | L210 A213 L211 A212 | L212 A216 L213 A215 | L214 A218 L215 A217 | L216 A220 L217 A219 | L218 A222 L219 A221 | L220 A224 L221 A223 | L222 A226 L223 A225
ref_plane "Work Plane1" through (0, -3.5, 0) normal (0, 1, 0) x (1, 0, 0)
mirror "Mirror1" about plane through (0, -3.5, 0) normal (0, 1, 0) of "Extrusion2"
body "Solid1"
